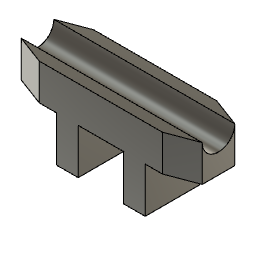
Yagi  v0 (Autodesk Fusion 360 design; units mm, degrees)
Autodesk Fusion 360 part; units mm, degrees
sketch "Sketch1" plane through (0, 0, 0) normal (0, 0, 1) x (1, 0, 0)
sketch "Sketch2" plane through (0, 0, 0) normal (0, 0, 1) x (1, 0, 0)
  line L0 (-5, -5) -> (95, -5)
  line L1 (95, -5) -> (95, 13)
  line L2 (95, 13) -> (-5, 13)
  line L3 (-5, 13) -> (-5, -5)
  line L4 (-5, 13) -> (11, 13)
  line L5 (95, 13) -> (79, 13)
  line L6 (11, 13) -> (79, 13)
  line L7 (79, 13) -> (79, 19)
  line L8 (79, 19) -> (11, 19)
  line L9 (11, 19) -> (11, 13)
  line L10 (11, -5) -> (79, -5)
  line L11 (79, -5) -> (79, -11)
  line L12 (79, -11) -> (11, -11)
  line L13 (11, -11) -> (11, -5)
  line L14 (11, -11) -> (-5, -5)
  line L15 (-5, 13) -> (11, 19)
  line L16 (79, 19) -> (95, 13)
  line L17 (95, -5) -> (79, -11)
  dimension "d1" = 100
  dimension "d2" = 18
  dimension "d3" = 16
  dimension "d4" = 16
  dimension "d5" = 68
  dimension "d6" = 6
  dimension "d7" = 68
  dimension "d8" = 6
  constraint horizontal L0
  constraint vertical L1
  constraint horizontal L2
  constraint vertical L3
  constraint horizontal L4
  constraint horizontal L5
  constraint horizontal L6
  constraint vertical L7
  constraint horizontal L8
  constraint vertical L9
  constraint horizontal L10
  constraint vertical L11
  constraint horizontal L12
  constraint vertical L13
  constraint coincident L0 L10.start
  measures "d1" distance of L0.start L0.end
  measures "d2" distance of L0.start L2.end
  measures "d3" distance of L2.end L4.end
  measures "d4" distance of L1.end L5.end
  measures "d5" distance of L4.end L5.end
  measures "d6" distance of L4.end L8.end
  measures "d7" distance of L10.start L10.end
  measures "d8" distance of L10.start L12.end
extrude "Extrude1" add sketch "Sketch2" along normal blind 20
sketch "Sketch3" plane through (95, 0, 0) normal (1, 0, 0) x (0, 1, 0)
  line L0 (-5, 0) -> (13, 0)
  line L1 (13, 0) -> (13, 20)
  line L2 (13, 20) -> (-5, 20)
  line L3 (-5, 20) -> (-5, 0)
  line L4 (-5, 20) -> (4, 20)
  arc A0 (-5, 20) -> (13, 20) centre (4, 20) ccw
  dimension "d11" = 9
  dimension "d12" = 18
  constraint coincident L2.end L3.start
  constraint perpendicular L1 L4
  constraint coincident L4.end A0.centre
  measures "d11" distance of L2.end L4.end
  measures "d12" diameter of A0
extrude "Extrude2" cut sketch "Sketch3" against normal blind 100 contours L2 L4 A0
sketch "Sketch4" plane through (0, 0, 0) normal (0, 0, 1) x (1, 0, 0)
  line L0 (79, -11) -> (69.5, -11)
  line L1 (69.5, -11) -> (69.5, 19)
  line L2 (69.5, 19) -> (79, 19)
  line L3 (79, 19) -> (79, -11)
  line L4 (11, -11) -> (20.5, -11)
  line L5 (20.5, -11) -> (20.5, 19)
  line L6 (20.5, 19) -> (11, 19)
  line L7 (11, 19) -> (11, -11)
  line L8 (20.5, -11) -> (32.5, -11)
  line L9 (32.5, -11) -> (32.5, 19)
  line L10 (32.5, 19) -> (20.5, 19)
  line L11 (20.5, 19) -> (20.5, -11)
  line L12 (69.5, -11) -> (57.5, -11)
  line L13 (57.5, -11) -> (57.5, 19)
  line L14 (57.5, 19) -> (69.5, 19)
  line L15 (69.5, 19) -> (69.5, -11)
  dimension "d15" = 9.5
  dimension "d16" = 30
  dimension "d17" = 9.5
  dimension "d18" = 30
  dimension "d19" = 12
  dimension "d20" = 30
  dimension "d21" = 12
  dimension "d22" = 30
  constraint horizontal L0
  constraint vertical L1
  constraint horizontal L2
  constraint vertical L3
  constraint horizontal L4
  constraint vertical L5
  constraint horizontal L6
  constraint vertical L7
  constraint horizontal L8
  constraint vertical L9
  constraint horizontal L10
  constraint vertical L11
  constraint horizontal L12
  constraint vertical L13
  constraint horizontal L14
  constraint vertical L15
  measures "d15" distance of L0.start L0.end
  measures "d16" distance of L0.start L2.end
  measures "d17" distance of L4.start L4.end
  measures "d18" distance of L4.start L6.end
  measures "d19" distance of L4.end L8.end
  measures "d20" distance of L4.end L5.end
  measures "d21" distance of L0.end L12.end
  measures "d22" distance of L0.end L1.end
extrude "Extrude3" add sketch "Sketch4" against normal blind 25 contours L1 L12 L13 L14 L15 | L5 L8 L9 L10 L11
